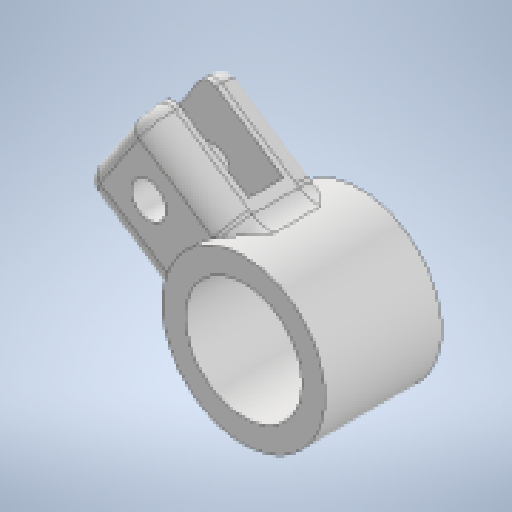
# Autodesk Inventor part: CAR_HOLDER
Saved by Autodesk Inventor 2025.4 (Build 294407000, 407)
## iProperties
Created: 2026-07-12
Part Number: CAR_HOLDER
Material: 常规
Document SubType Name: Modeling
Designer: Admin
Density: 1 g/cm^3
Appearance: 默认
Author: Admin
Autodesk Inventor part; units mm, degrees
ref_plane "YZ Plane" through (0, 0, 0) normal (1, 0, 0) x (0, 1, 0)
ref_plane "XZ Plane" through (0, 0, 0) normal (0, 1, 0) x (-1, 0, 0)
ref_plane "XY Plane" through (0, 0, 0) normal (0, 0, 1) x (1, 0, 0)
sketch "草图1" plane through (0, 0, 0) normal (0, 0, 1) x (1, 0, 0)
  circle A0 centre (9.511034, -5.491198) radius 5
  circle A1 centre (9.511034, -5.491198) radius 7
  point P0 (0, 0)
  dimension "d0" = 14
  constraints: 1 centre point, 1 coincident
  measures "d0" diameter of A1
extrude "拉伸1" add sketch "草图1" along normal mid plane 10
sketch "草图2" plane through (0, 0, 0) normal (0, 0, 1) x (1, 0, 0)
  circle A0 centre (-18.412784, 13.015838) radius 33.5
  circle A1 centre (9.511034, -5.491198) radius 7
  line L0 (-18.412784, 13.015838) -> (9.511034, -5.491198)
  circle A2 centre (0.342019, 0.585739) radius 1.5
  line L1 (-18.412784, 13.015838) -> (4.509753, -2.176505)
  line L2 (1.747509, -6.344239) -> (7.271998, 1.991229)
  line L3 (7.271998, 1.991229) -> (-0.229923, 6.963269)
  line L4 (-0.229923, 6.963269) -> (-5.754412, -1.372199)
  line L5 (-5.754412, -1.372199) -> (1.747509, -6.344239)
  arc A3 (7.271998, 1.991229) -> (9.103851, 1.496949) centre (8.929344, 4.491869) ccw
  arc A4 (2.916424, -7.838775) -> (1.747509, -6.344239) centre (0.090163, -8.84488) ccw
  point P0 (0, 0)
  point P1 (4.509753, -2.176505)
  dimension "d3" = 3
  dimension "d6" = 10
  dimension "d7" = 27.5
  dimension "d17" = 33.5
  dimension "d18" = 11
  dimension "d19" = 4
  constraints: 12 end point, 6 point on circle, 4 tangent, 3 centre point, 3 point on line, 2 parallel, 2 perpendicular, 1 midpoint
  measures "d3" diameter of A2
  measures "d6" distance of L2.start L2.end
  measures "d7" distance from line of L0.start L2
  measures "d17" distance of L0.end L0.start
  measures "d18" distance of L0.end A2.centre
  measures "d19" distance from line of L4 A2.centre
extrude "拉伸2" add sketch "草图2" along normal mid plane 8 contours A4 L2 A1 | A1 L2 A3 | L2 L5 L4 L0 A2 A1 | A1 L0 A2 L4 L3 L2
sketch "草图3" plane through (-0.229923, 6.963269, 4) normal (0.5524488, 0.8335468, 0) x (0.8335468, -0.5524488, 0)
  line L0 (5.5, 0) -> (2.5, 0)
  line L1 (2.5, 0) -> (2.5, 3.092497)
  line L2 (9, 0) -> (0, 0)
  line L3 (5.5, 0) -> (5.5, 3.092497)
  line L4 (0, 8) -> (0, 0)
  line L5 (0, 2.5) -> (8, 2.5)
  line L6 (8, 2.5) -> (8, 5.5)
  line L7 (8, 5.5) -> (0, 5.5)
  line L8 (0, 5.5) -> (0, 2.5)
  point P0 (4.038502, 4)
  point P1 (0, 5.5)
  dimension "d11" = 3
  dimension "d13" = 2.5
  dimension "d20" = 2.5
  constraints: 12 end point, 3 perpendicular, 2 parallel, 2 point on line, 1 coincident, 1 horizontal, 1 vertical
  measures "d11" distance between parallel lines of L7 L5
  measures "d13" distance between parallel lines of L2 L5
  measures "d20" distance between parallel lines of L6 L3
extrude "拉伸3" cut sketch "草图3" along normal through all both and the other way through all contours L5 L4 L7 L6
fillet "圆角1" radius 2 8 edges at (2.4532, -6.9967, -4) (-2.0035, -3.8582, -4) (8.1478, 1.5955, -4) (3.521, 4.4772, -4) (8.1478, 1.5955, 4) (3.521, 4.4772, 4) (2.4532, -6.9967, 4) (-2.0035, -3.8582, 4)
fillet "圆角2" radius 1 5 edges at (-5.4308, -0.8839, 3.4142) (-5.7544, -1.3722, 1.75) (-0.5535, 6.475, 3.4142) (-0.2299, 6.9633, 1.75) (-2.9922, 2.7955, 4)
fillet "圆角3" radius 1 5 edges at (-0.5535, 6.475, -3.4142) (-0.2299, 6.9633, -1.75) (-5.4308, -0.8839, -3.4142) (-5.7544, -1.3722, -1.75) (-2.9922, 2.7955, -4)
